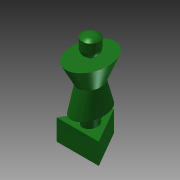
# Autodesk Inventor part: femsle
Saved by Autodesk Inventor 2015 (Build 190159000, 159)
## iProperties
Created: 2018-01-04
Part Number: femsle
Material: PMMA Plastic
Document SubType Name: Modeling
Designer: Administrator
Density: 1.188 g/cm^3
Appearance: Smooth - Dark Forest Green
Mass: 3.80659 g
Surface Area: 18.6026 cm^2
Volume: 3.2042 cm^3
Author: Administrator
Autodesk Inventor part; units mm, degrees
sketch "Sketch1" plane through (0, 0, 0) normal (0, 1, 0) x (-1, 0, 0)
  line L0 (0, 0) -> (16.3071, 0)
  line L1 (16.3071, 0) -> (8.1536, -14.1224)
  line L2 (8.1536, -14.1224) -> (0, 0)
  point P0 (8.1536, 0)
  dimension "d1" = 14.1224
  dimension "d3" = 0
  constraints: 6 end point, 1 equal length, 1 horizontal, 1 midpoint
  measures "d1" vertical distance of L0.end L1.end
  measures "d3" horizontal distance of L1.end point (8.154, 0)
extrude "Extrusion1" add sketch "Sketch1" along normal blind 8.128
sketch "Sketch2" plane through (0, 8.128, 0) normal (0, 1, 0) x (1, 0, 0)
  ellipse E0 centre (-7.9375, 4.7625) end of major axis (-5.2705, 4.7625) minor radius 3.175
  line L0 (-16.3071, 0) -> (0, 0) projected
  line L1 (0, 0) -> (-8.1536, 14.1224) projected
  line L2 (-8.1536, 14.1224) -> (-16.3071, 0) projected
  line L3 (-8.1536, 14.1224) -> (-16.3071, 0) projected
  dimension "d8" = 2.667
  dimension "d9" = 3.175
  constraints: 2 other
ref_plane "Work Plane1" through (0, 12.954, 0) normal (0, 1, 0) x (1, 0, 0)
sketch "Sketch3" plane through (0, 12.954, 0) normal (0, 1, 0) x (1, 0, 0)
  ellipse E0 centre (-7.9375, 4.7625) end of major axis (-7.9375, 8.3185) minor radius 2.794
  point P0 (0, 0)
  dimension "d11" = 2.794
  dimension "d12" = 3.556
  dimension "d13" = 0
  dimension "d14" = 0
  constraints: 2 other
  measures "d13" distance of point (-7.938, 4.763) point (-7.938, 4.763)
  measures "d14" distance of point (-7.938, 4.763) point (-7.938, 4.763)
loft "Loft1" add profiles "Sketch3", "Sketch2" contours all / E0
ref_plane "Work Plane2" through (-7.9375, 22.098, -4.7625) normal (0, 1, 0) x (1, 0, 0)
sketch "Sketch4" plane through (-7.9375, 22.098, -4.7625) normal (0, 1, 0) x (1, 0, 0)
  ellipse E0 centre (0, 0) end of major axis (0, 4.953) minor radius 3.937
  point P0 (7.9375, -4.7625)
  dimension "d20" = 3.937
  dimension "d21" = 4.953
  constraints: 2 other
sketch "Sketch5" plane through (-7.9375, 12.954, -4.7625) normal (0, 1, 0) x (1, 0, 0)
  ellipse E0 centre (0, 0) end of major axis (0, -7.62) minor radius 5.08
  point P0 (7.9375, -4.7625)
  dimension "d22" = 5.08
  dimension "d23" = 7.62
  constraints: 2 other
loft "Loft2" add profiles "Sketch5", "Sketch4"
ref_plane "Work Plane3" through (-7.9375, 30.734, -4.7625) normal (0, 1, 0) x (1, 0, 0)
sketch "Sketch7" plane through (-7.9375, 30.734, -4.7625) normal (0, 1, 0) x (1, 0, 0)
  ellipse E0 centre (0, 0) end of major axis (0, 9.652) minor radius 6.858
  point P0 (7.9375, -4.7625)
  dimension "d29" = 6.858
  dimension "d30" = 9.652
  constraints: 2 other
loft "Loft3" add profiles "Sketch7" section 1 edges at (-4.0005, 22.098, -4.7625) (-11.8745, 22.098, -4.7625)
sketch "Sketch8" plane through (-7.9375, 30.734, -4.7625) normal (0, 1, 0) x (1, 0, 0)
  ellipse E0 centre (0, 0) end of major axis (0, -9.652) minor radius 6.858 projected
  line L0 (0, 9.652) -> (0, -9.652)
  point P0 (7.9375, -4.7625)
  constraints: 2 end point, 1 vertical, 3 other
ref_plane "Work Plane4" through (-7.9375, 30.734, -14.4145) normal (-1, 0, 0) x (0, 0, 1)
sketch "Sketch9" plane through (-7.9375, 30.734, -14.4145) normal (-1, 0, 0) x (0, 0, 1)
  line L0 (0, 0) -> (19.304, 0) projected
  line L1 (9.652, 0) -> (9.652, 7.4025)
  line L2 (6.35, 6.35) -> (6.35, 3.0298)
  arc A0 (9.652, 7.4025) -> (6.35, 6.35) centre (9.1003, 3.4274) ccw
  arc A1 (6.35, 3.0298) -> (9.652, 0) centre (9.391, 3.0298) ccw
  point P0 (14.4145, -30.734)
  constraints: 4 end point, 4 point on circle, 2 centre point, 2 vertical, 1 midpoint, 1 tangent
revolve "Revolution1" add sketch "Sketch9" angle 360 about axis through (-7.9375, 30.734, -4.7625) along (0, 1, 0)
body "Solid1"
